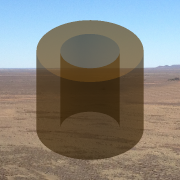
# Autodesk Inventor part: ductFan
Saved by Autodesk Inventor 2014 SP1 (Build 180222100, 222)
## iProperties
Created: 2014-05-22
Part Number: ductFan
Material: Polycarbonate, Smoke
Document SubType Name: Modeling
Designer: Dave
Mass: 6919.11 g
Surface Area: 2837.56 cm^2
Volume: 5765.93 cm^3
Density: 1.2 g/cm^3
Appearance: Polycarbonate - Smoked
Author: Dave
Autodesk Inventor part; units mm, degrees
ref_plane "YZ Plane" through (0, 0, 0) normal (1, 0, 0) x (0, 1, 0)
ref_plane "XZ Plane" through (0, 0, 0) normal (0, 1, 0) x (-1, 0, 0)
ref_plane "XY Plane" through (0, 0, 0) normal (0, 0, 1) x (1, 0, 0)
sketch "Sketch1" plane through (0, 0, 0) normal (0, 1, 0) x (-1, 0, 0)
  circle A0 centre (0.5253, 0) radius 114.3
  circle A1 centre (0.5253, 0) radius 63.5
  point P0 (0, 0)
  dimension "d0" = 228.6
  dimension "d1" = 50.8
  constraints: 2 centre point
  measures "d0" diameter of A0
  measures "d1" radial gap between concentric circles of A1 A0
extrude "Extrusion1" add sketch "Sketch1" along normal blind 203.2
body "Solid1"
